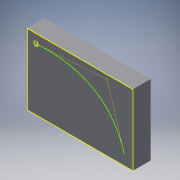
# Autodesk Inventor part: Rectangular Pattern Curve
Saved by Autodesk Inventor 2016 (Build 200138000, 138)
## iProperties
Created: 2013-12-12
Part Number: Rectangular Pattern Curve
Material: Generic
Document SubType Name: Modeling
Designer: John
Density: 1 g/cm^3
Appearance: Default
Author: John
Autodesk Inventor part; units mm, degrees
ref_plane "YZ Plane" through (0, 0, 0) normal (1, 0, 0) x (0, 1, 0)
ref_plane "XZ Plane" through (0, 0, 0) normal (0, 1, 0) x (-1, 0, 0)
ref_plane "XY Plane" through (0, 0, 0) normal (0, 0, 1) x (1, 0, 0)
sketch "Sketch1" plane through (0, 0, 0) normal (0, 0, 1) x (1, 0, 0)
  line L0 (0, 0) -> (152.4, 0)
  line L1 (152.4, 0) -> (152.4, 101.6)
  line L2 (152.4, 101.6) -> (0, 101.6)
  line L3 (0, 101.6) -> (0, 0)
  dimension "d0" = 152.4
  dimension "d1" = 101.6
  constraints: 8 end point, 2 parallel, 1 horizontal, 1 perpendicular
  measures "d0" distance of L2.end L1.end
  measures "d1" distance of L1.end L0.end
extrude "Extrusion1" add sketch "Sketch1" along normal blind 25.4
sketch "Sketch2" plane through (0, 0, 25.4) normal (0, 0, 1) x (1, 0, 0)
  line L0 (152.4, 101.6) -> (0, 101.6) projected
  line L1 (0, 101.6) -> (0, 0) projected
  circle A0 centre (12.7, 88.9) radius 3.175
  dimension "d4" = 6.35
  dimension "d5" = 12.7
  dimension "d6" = 12.7
  constraints: 1 centre point
  measures "d4" diameter of A0
  measures "d5" distance from line of L1 A0.centre
  measures "d6" distance from line of L0 A0.centre
extrude "Extrusion2" cut sketch "Sketch2" against normal through all
sketch "Sketch3" plane through (0, 0, 25.4) normal (0, 0, 1) x (1, 0, 0)
  circle A0 centre (12.7, 88.9) radius 3.175 projected
  line L0 (0, 0) -> (152.4, 0) projected
  line L1 (152.4, 0) -> (152.4, 101.6) projected
  line L2 (152.4, 101.6) -> (0, 101.6) projected
  line L3 (0, 101.6) -> (0, 0) projected
  line L4 (12.7, 88.9) -> (115.5228, 95.2014) construction
  line L5 (115.5228, 95.2014) -> (139.9001, 15.1047) construction
  spline S0 degree 2 poles (12.7, 88.9) (115.5228, 95.2014) (139.9001, 15.1047) knots 1 1 1 2 2 2
  constraints: 3 other
body "Solid1"
